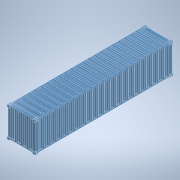
# Autodesk Inventor part: ContainerV1
Saved by Autodesk Inventor 2022.3 (Build 263350030, 350C)
## iProperties
Created: 2022-08-11
Part Number: ContainerV1
Material: Aluminium 5005-H18
Document SubType Name: Modeling
Designer: syniawa
Density: 2.7 g/cm^3
Appearance: Dunkelcyan
Author: syniawa
Autodesk Inventor part; units mm, degrees
sketch "Skizze1" plane through (0, 0, 0) normal (0, 1, 0) x (-1, 0, 0)
  line L0 (3795.2248, 4653.172) -> (1355.2248, 4653.172)
  line L1 (1355.2248, 4653.172) -> (1355.2248, -7536.828)
  line L2 (1355.2248, -7536.828) -> (3795.2248, -7536.828)
  line L3 (3795.2248, -7536.828) -> (3795.2248, 4653.172)
  point P0 (0, 0)
  dimension "d0" = 12190
  dimension "d1" = 2440
  constraints: 8 end point, 2 horizontal, 2 parallel, 1 perpendicular, 1 vertical
  measures "d0" distance of L2.end L0.start
  measures "d1" distance of L1.end L2.end
extrude "Extrusion1" add sketch "Skizze1" along normal blind 2590
sketch "Skizze2" plane through (-1355.2248, 0, 4653.172) normal (1, 0, 0) x (0, 0, -1)
  line L0 (-50, 2640) -> (250, 2640)
  line L1 (250, 2640) -> (250, 2440)
  line L2 (250, 2440) -> (-50, 2440)
  line L3 (-50, 2440) -> (-50, 2640)
  line L4 (0, 2590) -> (12190, 2590) projected
  line L5 (0, 0) -> (0, 2590) projected
  point P0 (4653.172, 0)
  dimension "d4" = 200
  dimension "d5" = 300
  dimension "d6" = 50
  dimension "d7" = 50
  constraints: 8 end point, 2 parallel, 1 horizontal, 1 perpendicular
  measures "d4" distance of L2.end L0.start
  measures "d5" distance of L0.start L0.end
  measures "d6" distance between parallel lines of L4 L0
  measures "d7" distance between parallel lines of L5 L3
extrude "Extrusion2" add sketch "Skizze2" along normal blind 20 and the other way blind 200
sketch "Skizze3" plane through (-1555.2248, 2440, 4703.172) normal (0, 0, 1) x (1, 0, 0)
  line L0 (110, 170) -> (110, 170)
  line L1 (160, 120) -> (160, 80)
  line L2 (110, 30) -> (110, 30)
  line L3 (60, 80) -> (60, 120)
  line L4 (220, 200) -> (0, 200) projected
  line L5 (0, 0) -> (220, 0) projected
  line L6 (0, 0) -> (0, 200) projected
  arc A0 (110, 170) -> (60, 120) centre (110, 120) ccw
  arc A1 (160, 120) -> (110, 170) centre (110, 120) ccw
  arc A2 (110, 30) -> (160, 80) centre (110, 80) ccw
  arc A3 (60, 80) -> (110, 30) centre (110, 80) ccw
  point P0 (1555.2248, -2440)
  point P1 (60, 170)
  point P2 (160, 170)
  point P3 (110, 170)
  point P4 (110, 30)
  dimension "d12" = 100
  dimension "d14" = 30
  dimension "d16" = 30
  dimension "d17" = 60
  dimension "d18" = 50
  constraints: 8 end point, 8 point on circle, 8 tangent, 4 centre point, 4 point on line, 3 equal radius, 2 parallel, 1 horizontal, 1 perpendicular
  measures "d12" distance of point (60, 170) point (160, 170)
  measures "d14" distance between parallel lines of L4 L0
  measures "d16" distance between parallel lines of L5 L2
  measures "d17" distance between parallel lines of L6 L3
  measures "d18" radius of A0
extrude "Extrusion3" cut sketch "Skizze3" against normal blind 20
sketch "Skizze4" plane through (-1335.2248, 0, 4653.172) normal (1, 0, 0) x (0, 0, -1)
  line L0 (90, 2610) -> (110, 2610)
  line L1 (150, 2570) -> (150, 2510)
  line L2 (110, 2470) -> (90, 2470)
  line L3 (50, 2510) -> (50, 2570)
  line L4 (-50, 2440) -> (250, 2440) projected
  line L5 (250, 2640) -> (-50, 2640) projected
  line L6 (-50, 2640) -> (-50, 2440) projected
  arc A0 (150, 2570) -> (110, 2610) centre (110, 2570) ccw
  arc A1 (90, 2610) -> (50, 2570) centre (90, 2570) ccw
  arc A2 (50, 2510) -> (90, 2470) centre (90, 2510) ccw
  arc A3 (110, 2470) -> (150, 2510) centre (110, 2510) ccw
  point P0 (4653.172, 0)
  point P1 (50, 2610)
  point P2 (150, 2610)
  dimension "d21" = 100
  dimension "d22" = 30
  dimension "d23" = 30
  dimension "d24" = 100
  dimension "d25" = 40
  constraints: 8 end point, 8 point on circle, 8 tangent, 4 centre point, 4 point on line, 3 equal radius, 2 parallel, 1 horizontal, 1 perpendicular
  measures "d21" distance of point (50, 2610) point (150, 2610)
  measures "d22" distance between parallel lines of L4 L2
  measures "d23" distance between parallel lines of L5 L0
  measures "d24" distance between parallel lines of L3 L6
  measures "d25" radius of A0
extrude "Extrusion5" cut sketch "Skizze4" against normal blind 20
sketch "Skizze5" plane through (-1555.2248, 2640, 4703.172) normal (0, 1, 0) x (1, 0, 0)
  line L0 (40, 40) -> (180, 40)
  line L1 (180, 40) -> (180, 260)
  line L2 (180, 260) -> (40, 260)
  line L3 (40, 260) -> (40, 40)
  line L4 (0, 0) -> (0, 300) projected
  line L5 (220, 300) -> (220, 0) projected
  line L6 (0, 300) -> (220, 300) projected
  line L7 (220, 0) -> (0, 0) projected
  point P0 (1555.2248, 4703.172)
  dimension "d30" = 40
  dimension "d31" = 40
  dimension "d32" = 40
  dimension "d33" = 40
  constraints: 8 end point, 2 parallel, 1 horizontal, 1 perpendicular
  measures "d30" distance between parallel lines of L4 L3
  measures "d31" distance between parallel lines of L5 L1
  measures "d32" distance between parallel lines of L6 L2
  measures "d33" distance between parallel lines of L7 L0
extrude "Extrusion6" cut sketch "Skizze5" against normal blind 50 contours L3 L2 L1 L0
pattern_linear "Rechteckige Anordnung2" count 2 spacing 12000 along (0, 0, -1) of "Extrusion6", "Extrusion5", "Extrusion3", "Extrusion2"
ref_plane "Arbeitsebene1" through (0, 1295, 0) normal (0, 1, 0) x (1, 0, 0)
ref_plane "Arbeitsebene2" through (-2575.2248, 2590, 4403.172) normal (1, 0, 0) x (0, 0, -1)
sketch "Skizze8" plane through (-3795.2248, 0, -7536.828) normal (-1, 0, 0) x (0, 0, 1)
  line L0 (0, 2590) -> (12190, 2590) projected
  line L1 (300, 2590) -> (400, 2510)
  line L2 (400, 2510) -> (550, 2510)
  line L3 (550, 2510) -> (650, 2590)
  line L4 (300, 2590) -> (650, 2590)
  line L5 (0, 0) -> (0, 2590) projected
  point P0 (7536.828, 0)
  dimension "d60" = 300
  dimension "d61" = 100
  dimension "d62" = 100
  dimension "d63" = 150
  dimension "d64" = 80
  constraints: 8 end point, 2 parallel, 2 point on line
  measures "d60" distance from line of L5 L1.start
  measures "d61" horizontal distance of L1.start L1.end
  measures "d62" horizontal distance of L3.end L2.end
  measures "d63" distance of L1.end L2.end
  measures "d64" distance between parallel lines of L0 L2
ref_plane "Arbeitsebene3" through (-3695.2248, 0, -7536.828) normal (-1, 0, 0) x (0, 0, 1)
ref_plane "Arbeitsebene4" through (-1455.2248, 0, 4653.172) normal (1, 0, 0) x (0, 0, -1)
extrude "Extrusion9" cut sketch "Skizze8" against normal up to surface (2240 mm away) from surface at -100
pattern_linear "Rechteckige Anordnung4" count 22 spacing 534 along (0, 0, 1) of "Extrusion9"
sketch "Skizze9" plane through (0, 2590, 0) normal (0, 1, 0) x (1, 0, 0)
  line L0 (-3795.2248, 7536.828) -> (-3795.2248, -4653.172) projected
  line L1 (-3795.2248, -4327.172) -> (-3715.2248, -4227.172)
  line L2 (-3715.2248, -4227.172) -> (-3715.2248, -4077.172)
  line L3 (-3695.2248, -4327.172) -> (-3695.2248, -4227.172) projected
  line L4 (-3715.2248, -4077.172) -> (-3795.2248, -3977.172)
  line L5 (-3795.2248, -3977.172) -> (-3795.2248, -4327.172)
  line L6 (-3795.2248, -4653.172) -> (-1555.2248, -4653.172) projected
  point P0 (0, 0)
  dimension "d72" = 326
  dimension "d73" = 100
  dimension "d74" = 150
  dimension "d75" = 100
  dimension "d76" = 80
  constraints: 8 end point, 2 parallel, 1 point on line
  measures "d72" distance from line of L6 L1.start
  measures "d73" vertical distance of L1.start L1.end
  measures "d74" distance of L1.end L2.end
  measures "d75" vertical distance of L4.end L2.end
  measures "d76" distance between parallel lines of L0 L2
ref_plane "Arbeitsebene5" through (0, 2490, 0) normal (0, 1, 0) x (1, 0, 0)
ref_plane "Arbeitsebene6" through (0, 100, 0) normal (0, -1, 0) x (1, 0, 0)
extrude "Extrusion10" cut sketch "Skizze9" against normal up to surface (2390 mm away) from surface at -100
pattern_linear "Rechteckige Anordnung5" count 22 spacing 534 along (0, 0, -1) of "Extrusion10"
mirror "Spiegeln3" about plane through (-2575.2248, 2590, 4403.172) normal (1, 0, 0) of "Extrusion10", "Rechteckige Anordnung5"
mirror "Spiegeln4" about plane through (0, 1295, 0) normal (0, 1, 0) of "Extrusion9", "Rechteckige Anordnung4"
mirror "Spiegeln5" about plane through (0, 1295, 0) normal (0, 1, 0) of "Extrusion6", "Extrusion5", "Extrusion3", "Extrusion2", "Rechteckige Anordnung2"
mirror "Spiegeln6" about plane through (-2575.2248, 2590, 4403.172) normal (1, 0, 0) of "Extrusion6", "Extrusion5", "Extrusion3", "Extrusion2", "Rechteckige Anordnung2", "Spiegeln5"
sketch "Skizze10" plane through (-1355.2248, 2590, 4403.172) normal (1, 0, 0) x (0, 0, -1)
  line L0 (-250, -2440) -> (-250, -150) projected
  line L1 (-250, -385) -> (-150, -485)
  line L2 (-150, -485) -> (-150, -635)
  line L3 (-150, -635) -> (-250, -735)
  line L4 (-250, -1120) -> (-150, -1220)
  line L5 (-150, -1220) -> (-150, -1370)
  line L6 (-150, -1370) -> (-250, -1470)
  line L7 (-250, -1855) -> (-170, -1955)
  line L8 (-170, -1955) -> (-170, -2105)
  line L9 (-170, -2105) -> (-250, -2205)
  line L10 (0, -2590) -> (11700, -2590) projected
  point P0 (4403.172, -2590)
  dimension "d84" = 150
  dimension "d85" = 100
  dimension "d86" = 100
  dimension "d88" = 150
  dimension "d89" = 100
  dimension "d90" = 100
  dimension "d91" = 150
  dimension "d92" = 100
  dimension "d93" = 100
  dimension "d94" = 80
  dimension "d95" = 100
  dimension "d96" = 385
  dimension "d97" = 385
  dimension "d98" = 385
  constraints: 18 end point, 8 point on line, 1 parallel, 1 perpendicular, 1 vertical
  measures "d84" distance of L1.end L2.end
  measures "d85" horizontal distance of L1.start L1.end
  measures "d86" horizontal distance of L2.end L3.end
  measures "d88" distance of L4.end L5.end
  measures "d89" horizontal distance of L4.start L4.end
  measures "d90" horizontal distance of L5.end L6.end
  measures "d91" distance of L7.end L8.end
  measures "d92" vertical distance of L7.start L7.end
  measures "d93" vertical distance of L9.end L8.end
  measures "d94" distance between parallel lines of L0 L8
  measures "d95" distance between parallel lines of L0 L5
  measures "d96" distance from line of L9.end L10
  measures "d97" distance of L6.end L7.start
  measures "d98" distance of L3.end L4.start
ref_plane "Arbeitsebene7" through (-1655.2248, 2590, 4403.172) normal (1, 0, 0) x (0, 0, -1)
ref_plane "Arbeitsebene8" through (-3495.2248, 0, -7296.828) normal (-1, 0, 0) x (0, 0, 1)
extrude "Extrusion12" cut sketch "Skizze10" against normal blind 770 from surface at -300
mirror "Spiegeln7" about plane through (-2575.2248, 2590, 4403.172) normal (1, 0, 0) of "Extrusion12"
sketch "Skizze11" plane through (0, 2590, 0) normal (0, 1, 0) x (1, 0, 0)
  circle A0 centre (-3275.2248, -4673.172) radius 30
  circle A1 centre (-2875.2248, -4673.172) radius 30
  line L0 (-2575.2248, 10081.6202) -> (-2575.2248, -7311.9258) projected
  line L1 (-3595.2248, -4653.172) -> (-1555.2248, -4653.172) projected
  point P0 (0, 0)
  point P1 (-2852.8641, -4653.172)
  point P2 (-2897.5854, -4653.172)
  dimension "d105" = 300
  dimension "d106" = 400
  dimension "d107" = 60
  dimension "d108" = 60
  dimension "d109" = 20
  dimension "d110" = 20
  constraints: 2 centre point
  measures "d105" distance from line of L0 A1.centre
  measures "d106" distance of A0.centre A1.centre
  measures "d107" diameter of A1
  measures "d108" diameter of A0
  measures "d109" distance from line of L1 A1.centre
  measures "d110" distance from line of A0.centre L1
extrude "Extrusion13" add sketch "Skizze11" against normal blind 2500 contours A0 L1 | L1 A0 | A1 L1 picked at (-2866.6673, -4675.3774)
mirror "Spiegeln8" about plane through (-2575.2248, 2590, 4403.172) normal (1, 0, 0) of "Extrusion13"
sketch "Skizze12" plane through (-1355.2248, 150, 4653.172) normal (0, 0, 1) x (1, 0, 0)
  line L0 (-1170, 2240) -> (-200, 2240)
  line L1 (-200, 2240) -> (-200, 50)
  line L2 (-200, 50) -> (-1170, 50)
  line L3 (-1170, 50) -> (-1170, 2240)
  line L4 (-140, 2290) -> (-1230, 2290)
  line L5 (-1230, 2290) -> (-1230, 0)
  line L6 (-1230, 0) -> (-140, 0)
  line L7 (-140, 0) -> (-140, 2290)
  line L8 (-1070, 1320) -> (-1070, 970) projected
  line L9 (-300, 5501.7121) -> (-300, -1150.2853) projected
  line L10 (-897.6393, 2440) -> (-542.3607, 2440) projected
  line L11 (-2240, -150) -> (-200, -150) projected
  point P0 (1355.2248, -150)
  dimension "d113" = 100
  dimension "d114" = 100
  dimension "d115" = 200
  dimension "d116" = 200
  dimension "d117" = 60
  dimension "d118" = 50
  dimension "d119" = 60
  dimension "d120" = 50
  constraints: 16 end point, 4 parallel, 2 horizontal, 2 perpendicular
  measures "d113" distance between parallel lines of L8 L3
  measures "d114" distance between parallel lines of L9 L1
  measures "d115" distance between parallel lines of L10 L0
  measures "d116" distance between parallel lines of L2 L11
  measures "d117" distance between parallel lines of L1 L7
  measures "d118" distance between parallel lines of L6 L2
  measures "d119" distance between parallel lines of L5 L3
  measures "d120" distance between parallel lines of L0 L4
extrude "Extrusion14" add sketch "Skizze12" along normal blind 10 contours L3 L2 L9 L6 L5 L4 L0 | L9 L4 L7 L6 L2 L1 L0
mirror "Spiegeln9" about plane through (-2575.2248, 2590, 4403.172) normal (1, 0, 0) of "Extrusion14"
sketch "Skizze13" plane through (-1355.2248, 150, 4653.172) normal (0, 0, 1) x (1, 0, 0)
  line L0 (-80, 2340) -> (-80, -50) projected
  line L1 (-260, 1928) -> (-80, 1928)
  line L2 (-80, 1928) -> (-80, 1808)
  line L3 (-80, 1808) -> (-260, 1808)
  line L4 (-260, 1808) -> (-260, 1928)
  line L5 (-260, 1446) -> (-80, 1446)
  line L6 (-80, 1446) -> (-80, 1326)
  line L7 (-80, 1326) -> (-260, 1326)
  line L8 (-260, 1326) -> (-260, 1446)
  line L9 (-260, 964) -> (-80, 964)
  line L10 (-80, 964) -> (-80, 844)
  line L11 (-80, 844) -> (-260, 844)
  line L12 (-260, 844) -> (-260, 964)
  line L13 (-260, 482) -> (-80, 482)
  line L14 (-80, 482) -> (-80, 362)
  line L15 (-80, 362) -> (-260, 362)
  line L16 (-260, 362) -> (-260, 482)
  line L17 (-200, 0) -> (20, 0) projected
  point P0 (1355.2248, -150)
  point P1 (-80, 362)
  point P2 (-80, 482)
  point P3 (-80, 844)
  point P4 (-80, 964)
  point P5 (-80, 1326)
  point P6 (-80, 1446)
  point P7 (-80, 1928)
  dimension "d123" = 120
  dimension "d124" = 180
  dimension "d125" = 120
  dimension "d126" = 180
  dimension "d127" = 120
  dimension "d128" = 120
  dimension "d129" = 362
  dimension "d130" = 362
  dimension "d131" = 362
  dimension "d132" = 362
  constraints: 32 end point, 8 parallel, 6 point on line, 4 horizontal, 4 perpendicular
  measures "d123" distance between parallel lines of L13 L15
  measures "d124" distance of L14.end L15.end
  measures "d125" distance between parallel lines of L9 L11
  measures "d126" distance of L6.end L7.end
  measures "d127" distance between parallel lines of L7 L5
  measures "d128" distance of L1.end L2.end
  measures "d129" distance between parallel lines of L15 L17
  measures "d130" distance between parallel lines of L11 L13
  measures "d131" distance between parallel lines of L7 L9
  measures "d132" distance between parallel lines of L3 L5
extrude "Extrusion15" add sketch "Skizze13" along normal blind 15
mirror "Spiegeln10" about plane through (-2575.2248, 2590, 4403.172) normal (1, 0, 0) of "Extrusion15"
sketch "Skizze14" plane through (-1355.2248, 150, 4663.172) normal (0, 0, 1) x (1, 0, 0)
  line L0 (-1300, 1245) -> (-1140, 1245)
  line L1 (-1140, 1245) -> (-1140, 1145)
  line L2 (-1140, 1145) -> (-1300, 1145)
  line L3 (-1300, 1145) -> (-1300, 1245)
  line L4 (-1170, 50) -> (-1170, 2240) projected
  line L5 (-1270, 50) -> (-1270, 2240) projected
  line L6 (-2240, 0) -> (-2460, 0) projected
  point P0 (1355.2248, -150)
  dimension "d135" = 30
  dimension "d136" = 30
  dimension "d137" = 100
  dimension "d138" = 1145
  constraints: 8 end point, 2 parallel, 1 horizontal, 1 perpendicular
  measures "d135" distance between parallel lines of L1 L4
  measures "d136" distance between parallel lines of L5 L3
  measures "d137" distance between parallel lines of L0 L2
  measures "d138" distance between parallel lines of L2 L6
extrude "Extrusion16" add sketch "Skizze14" along normal blind 15
sketch "Skizze15" plane through (0, 2590, 0) normal (0, 1, 0) x (1, 0, 0)
  line L0 (-1555.2248, 7536.828) -> (-3595.2248, 7536.828) projected
  line L1 (-3545.2248, 7536.828) -> (-3445.2248, 7456.828)
  line L2 (-3445.2248, 7456.828) -> (-3295.2248, 7456.828)
  line L3 (-3295.2248, 7456.828) -> (-3195.2248, 7536.828)
  line L4 (-3595.2248, 7296.828) -> (-3595.2248, 7596.828) projected
  line L5 (-3795.2248, 7296.828) -> (-3795.2248, -4403.172) projected
  point P0 (0, 0)
  dimension "d141" = 150
  dimension "d142" = 100
  dimension "d143" = 80
  dimension "d144" = 100
  dimension "d150" = 250
  constraints: 6 end point, 2 point on line, 1 parallel
  measures "d141" distance of L1.end L2.end
  measures "d142" horizontal distance of L2.end L3.end
  measures "d143" distance between parallel lines of L0 L2
  measures "d144" horizontal distance of L1.end L1.start
  measures "d150" distance from line of L5 L1.start
ref_plane "Arbeitsebene9" through (0, 2490, 0) normal (0, 1, 0) x (1, 0, 0)
ref_plane "Arbeitsebene10" through (0, 100, 0) normal (0, -1, 0) x (1, 0, 0)
extrude "Extrusion17" cut sketch "Skizze15" against normal up to surface (2390 mm away) from surface at -100
pattern_linear "Rechteckige Anordnung6" count 4 spacing 534 along (1, 0, 0) of "Extrusion17"
move or copy body "Körper verschieben1" bodies to move or copy 1 copy no rotation origin (0, 0, 0) rotation axis (0, 1, 0) rotation angle 180
